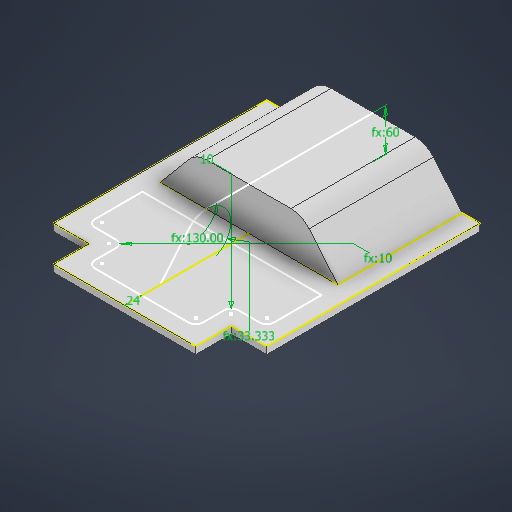
# Autodesk Inventor part: cap2
Saved by Autodesk Inventor 2027 (Build 310192060, 192F)
## iProperties
Created: 2026-07-29
Part Number: cap2
Material: 일반
Document SubType Name: Modeling
Designer: duqck
Density: 1 g/cm^3
Appearance: 기본값
Author: duqck
Autodesk Inventor part; units mm, degrees
ref_plane "YZ Plane" through (0, 0, 0) normal (1, 0, 0) x (0, 1, 0)
ref_plane "XZ Plane" through (0, 0, 0) normal (0, 1, 0) x (-1, 0, 0)
ref_plane "XY Plane" through (0, 0, 0) normal (0, 0, 1) x (1, 0, 0)
sketch "스케치1" plane through (0, 0, 0) normal (0, 1, 0) x (-1, 0, 0)
  line L0 (-150, 125) -> (-150, -175)
  line L1 (-150, -175) -> (150, -175)
  line L2 (150, -175) -> (150, 125)
  line L3 (150, 125) -> (100, 125)
  line L4 (100, 125) -> (100, 175)
  line L5 (100, 175) -> (-100, 175)
  line L6 (-100, 175) -> (-100, 125)
  line L7 (-100, 125) -> (-150, 125)
  point P0 (0, 0)
  dimension "d3" = 300
  dimension "d4" = 150
  dimension "d8" = 350
  dimension "d10" = 175
  dimension "d11" = 50
  constraints: 16 end point, 5 perpendicular, 3 equal length, 1 collinear, 1 vertical
  measures "d3" distance of L0.end L1.end
  measures "d4" distance from line of point (0, 0) L2
  measures "d8" distance between parallel lines of L5 L1
  measures "d10" distance from line of L5 point (0, 0)
  measures "d11" distance of L2.end L3.end
extrude "돌출1" add sketch "스케치1" along normal blind 10
sketch "스케치3" plane through (0, 0, 0) normal (0, 0, 1) x (1, 0, 0)
  line L0 (150, 10) -> (-150, 10) projected
  line L1 (-125, 10) -> (-84.6452, 58.0929)
  line L2 (-59.1104, 70) -> (59.1104, 70)
  line L3 (100, 0) -> (100, 10) projected
  line L4 (84.6452, 58.0929) -> (125, 10)
  line L5 (0, 0) -> (0, 70)
  arc A0 (-59.1104, 70) -> (-84.6452, 58.0929) centre (-59.1104, 36.6667) ccw
  arc A1 (84.6452, 58.0929) -> (59.1104, 70) centre (59.1104, 36.6667) ccw
  line L6 (125, 10) -> (-125, 10)
  point P0 (-74.654, 70)
  point P1 (74.654, 70)
  point P2 (125, 10)
  dimension "d15" = 130
  dimension "d17" = 33.3333
  dimension "d18" = 33.3333
  dimension "d19" = 300
  dimension "d22" = 250
  dimension "d24" = 60
  dimension "d25" = 0
  constraints: 10 end point, 4 point on circle, 4 point on line, 4 tangent, 2 centre point, 2 parallel, 2 symmetric about line, 1 midpoint, 1 perpendicular, 1 other
  measures "d15" angle of L1 L2
  measures "d17" radius of A0
  measures "d18" radius of A1
  measures "d19" distance of L0.start L0.end
  measures "d22" distance of L4.end L1.start
  measures "d24" distance between parallel lines of L6 L2
  measures "d25" distance between parallel lines of L0 L6
sketch "스케치4" plane through (0, 0, 0) normal (1, 0, 0) x (0, 1, 0)
  line L0 (70, -175) -> (70, 59.1104)
  line L1 (58.0929, 84.6452) -> (10, 125)
  line L2 (10, 175) -> (10, 125) projected
  line L3 (10, -175) -> (10, 125) projected
  line L4 (70, -175) -> (10, -175)
  arc A0 (70, 59.1104) -> (58.0929, 84.6452) centre (36.6667, 59.1104) ccw
  point P0 (0, 0)
  dimension "d27" = 130
  dimension "d28" = 33.3333
  dimension "d29" = 60
  constraints: 6 end point, 2 perpendicular, 2 point on circle, 2 tangent, 1 centre point
  measures "d27" angle of L1 L0
  measures "d28" radius of A0
  measures "d29" distance of L0.start L3.start
extrude "돌출3" add sketch "스케치3" against normal up to surface (175 mm away)
sketch "스케치5" plane through (0, 10, 0) normal (0, 1, 0) x (1, 0, 0)
  line L0 (125, 175) -> (125, 0) projected
  line L1 (125, 0) -> (-125, 0) projected
  line L2 (-125, 0) -> (-125, 175) projected
  line L3 (-125, 175) -> (-150, 175) projected
  line L4 (-150, 175) -> (-150, -125) projected
  line L5 (-150, -125) -> (-100, -125) projected
  line L6 (-100, -125) -> (-100, -175) projected
  line L7 (-100, -175) -> (100, -175) projected
  line L8 (100, -175) -> (100, -125) projected
  line L9 (100, -125) -> (150, -125) projected
  line L10 (150, -125) -> (150, 175) projected
  line L11 (150, 175) -> (125, 175) projected
  line L12 (66, -151) -> (-66, -151)
  line L13 (-76, -141) -> (-76, -111)
  line L14 (-86, -101) -> (-116, -101)
  line L15 (-126, -91) -> (-126, -24)
  line L16 (-126, -24) -> (126, -24)
  line L17 (126, -24) -> (126, -91)
  line L18 (116, -101) -> (86, -101)
  line L19 (76, -111) -> (76, -141)
  arc A0 (86, -101) -> (76, -111) centre (86, -111) ccw
  arc A1 (-76, -111) -> (-86, -101) centre (-86, -111) ccw
  arc A2 (116, -101) -> (126, -91) centre (116, -91) ccw
  arc A3 (-126, -91) -> (-116, -101) centre (-116, -91) ccw
  arc A4 (-76, -141) -> (-66, -151) centre (-66, -141) ccw
  arc A5 (66, -151) -> (76, -141) centre (66, -141) ccw
  point P0 (0, 0)
  dimension "d34" = 24
  dimension "d35" = 10
  dimension "d36" = 10
  constraints: 16 end point, 12 point on circle, 12 tangent, 6 centre point, 4 equal radius, 7 other
  measures "d34" distance between parallel lines of L7 L12
  measures "d35" radius of A0
  measures "d36" radius of A1
equation "\"d4\" = 0.5 * d3"
equation "\"d10\" = 0.5 * d8"
equation "\"d17\" = 0.5 * d14"
equation "\"d18\" = d17"
equation "\"d22\" = 0.833333 * d19"
equation "\"d24\" = 0.2 * d19"
equation "\"d27\" = d15"
equation "\"d28\" = d17"
equation "\"d29\" = d24"
equation "\"d36\" = d35"
equation "\"d14\" = 0.333333 * d16"
equation "\"d16\" = 200"
